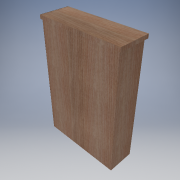
# Autodesk Inventor part: FrenteGrande
Saved by Autodesk Inventor 2016 (Build 200138000, 138)
## iProperties
Created: 2018-06-25
Part Number: FrenteGrande
Material: Wood (Birch)
Document SubType Name: Modeling
Designer: damia
Density: 0.55 g/cm^3
Appearance: Birch - Natural Polished
Mass: 3171.77 g
Surface Area: 8434.79 cm^2
Volume: 5766.85 cm^3
Author: damia
Autodesk Inventor part; units mm, degrees
ref_plane "YZ Plane" through (0, 0, 0) normal (1, 0, 0) x (0, 1, 0)
ref_plane "XZ Plane" through (0, 0, 0) normal (0, 1, 0) x (-1, 0, 0)
ref_plane "XY Plane" through (0, 0, 0) normal (0, 0, 1) x (1, 0, 0)
sketch "Sketch5" plane through (0, 0, 0) normal (0, 0, 1) x (1, 0, 0)
  line L0 (0, 0) -> (320, 0)
  line L1 (320, 0) -> (320, 150)
  line L2 (320, 150) -> (0, 150)
  line L3 (0, 150) -> (0, 0)
  dimension "d15" = 320
  dimension "d16" = 150
  constraints: 8 end point, 2 parallel, 1 horizontal, 1 perpendicular
  measures "d15" distance of L2.end L1.end
  measures "d16" distance of L0.end L1.end
extrude "Extrusion5" add sketch "Sketch5" along normal blind 18
sketch "Sketch6" plane through (0, 0, 0) normal (0, 0, -1) x (-1, 0, 0)
  line L0 (-312.3, 140) -> (-294.3, 140)
  line L1 (-294.3, 140) -> (-294.3, 5)
  line L2 (-294.3, 5) -> (-312.3, 5)
  line L3 (-312.3, 5) -> (-312.3, 140)
  line L4 (-320, 0) -> (-320, 150) projected
  line L5 (0, 0) -> (-320, 0) projected
  line L6 (-25.7, 140) -> (-7.7, 140)
  line L7 (-7.7, 140) -> (-7.7, 5)
  line L8 (-7.7, 5) -> (-25.7, 5)
  line L9 (-25.7, 5) -> (-25.7, 140)
  line L10 (0, 150) -> (0, 0) projected
  dimension "d19" = 18
  dimension "d20" = 135
  dimension "d21" = 7.7
  dimension "d22" = 5
  dimension "d23" = 18
  dimension "d24" = 7.7
  dimension "d25" = 5
  constraints: 16 end point, 4 parallel, 2 horizontal, 2 perpendicular, 1 horizontal alignment
  measures "d19" distance of L1.end L2.end
  measures "d20" distance of L0.end L1.end
  measures "d21" distance between parallel lines of L4 L3
  measures "d22" distance between parallel lines of L5 L2
  measures "d23" distance of L7.end L8.end
  measures "d24" distance between parallel lines of L10 L7
  measures "d25" distance between parallel lines of L5 L8
extrude "Extrusion6" add sketch "Sketch6" along normal blind 590
sketch "Sketch7" plane through (0, 0, -590) normal (0, 0, -1) x (-1, 0, 0)
  line L0 (-294.3, 140) -> (-294.3, 5) projected
  line L1 (-25.7, 5) -> (-25.7, 140) projected
  line L2 (-294.3, 140) -> (-25.7, 140)
  line L3 (-25.7, 140) -> (-25.7, 5)
  line L4 (-25.7, 5) -> (-294.3, 5)
  line L5 (-294.3, 5) -> (-294.3, 140)
  point P0 (0, 0)
  constraints: 8 end point, 2 parallel, 1 horizontal, 1 perpendicular
extrude "Extrusion7" add sketch "Sketch7" against normal blind 18
sketch "Sketch8" plane through (7.7, 5, -590) normal (0, -1, 0) x (1, 0, 0)
  line L0 (304.6, 590) -> (286.6, 590) projected
  line L1 (304.6, 590) -> (304.6, 0) projected
  line L2 (0, 0) -> (304.6, 0) projected
  line L3 (0, 590) -> (0, 0) projected
  line L4 (18, 590) -> (0, 590) projected
  line L5 (18, 590) -> (18, 18) projected
  line L6 (286.6, 18) -> (18, 18) projected
  line L7 (286.6, 590) -> (286.6, 18) projected
  line L8 (312.3, 590) -> (-7.7, 590) projected
extrude "Extrusion8" add sketch "Sketch8" against normal blind 9 contours L7 L6 L5 L8
equation "\"d16\" = Cajon02Altura"
equation "\"d24\" = d21"
equation "\"d25\" = d22"
equation "\"Cajon02Altura\" = 150"
body "Solid2"
